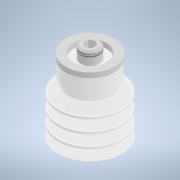
# Autodesk Inventor part: 189401 ESS-20-CS
Saved by Autodesk Inventor 2021 (Build 250183000, 183)
## iProperties
Created: 2026-04-25
Part Number: 189401 ESS-20-CS
Material: Generic
Catalog Web Link: www.3dfindit.com
Description: ESS-...-C-Suction cup complete
Vendor: FESTO
Document SubType Name: Modeling
Designer: psAdmin
Manufacturer: FESTO
Mass: 6.9 g
Surface Area: 38.5518 cm^2
Volume: 1.64725 cm^3
Density: 1 g/cm^3
Appearance: PSOLRGB-242-242-242
Category: PARTsolutions
Company: FESTO
Title: 189401 ESS-20-CS
Author: Cadenas PARTsolutions
Comments: Suction cup complete
PSOL_IDENT_0: {$CADENAS_DATA/23d-libs/festo/parts/e/ess/ess_c.prj},175 {VTYP=3D},{NB=189401 ESS-20-CS},{LINA=18940
PSOL_IDENT_1: 1 ESS-20-CS},{NN=ESS-...-C},{DATE=17.07.2025 08:23:31},{GEOMDATE=17.07.2025 08:23:17},{VERSION=},{LI
PSOL_IDENT_2: NEID=90},{WBVAR=},{WBNUMERIC=}  {NB=189401 ESS-20-CS},{LINA=189401 ESS-20-CS},{KT=2},{TNR=189401},{T
PSOL_IDENT_3: YP=ESS-20},{IDCODE=ESS-20-CS},{V=2.000},{MAT=CS},{COLOR=0.95,0.95,0.95,0.00},{MATN=15},{D1=20.000},{
PSOL_IDENT_4: D=3.000},{D2=15.000},{D3=15.500},{L1=23.000},{L2=2.400},{L3=16.400},{M=M6x1},{H=7.000},{M1=6.000},{Z
PSOL_IDENT_5: Z=0.1},{GR=4},{NENN=20},{GEO=2.000},{SDMN=20},{CNSMASSEXACT=0.00690},{GTIN=4052568042639},{REACH=Ja}
PSOL_IDENT_6: ,{REACHSVHC=Ja},{REACHHAZSUBS=7439-92-1},{REACHSCIP=a2c161a8-3d92-4cb1-8bd3-c3b2d55e9e9f},{REACHVALD
PSOL_IDENT_7: ATE=05.03.2025}
NB: 189401 ESS-20-CS
NN: ESS-...-C
NT: Suction cup complete
NBSYN: $TNR. $TYP.-$MAT.
LINA: 189401 ESS-20-CS
CATALOG: Festo
TNR: 189401
TYP: ESS-20
D1: 20
D: 3
D2: 15
D3: 15.5
L1: 23
L2: 2.4
L3: 16.4
M: M6x1
H: 7
CNSMASSEXACT: 0.0069
GTIN: 4052568042639
REACH: Yes
REACHSVHC: Yes
REACHHAZSUBS: 7439-92-1
REACHVALDATE: 05.03.2025
SUPPLIER: FESTO
ARTICLENO: 189401 ESS-20-CS
BOMINFO: 189401 ESS-20-CS
CREATOR: CADENAS GmbH
Autodesk Inventor part; units mm, degrees
sketch "Sketch_1" plane through (0, 0, 0) normal (0, 0, 1) x (1, 0, 0)
  line L0 (0, 16.0172) -> (0, 25.4)
  line L1 (0, 25.4) -> (2.3865, 25.4)
  line L2 (2.3865, 25.4) -> (3, 24.7865)
  line L3 (3, 24.7865) -> (3, 21.4)
  line L4 (3, 21.4) -> (5.25, 21.4)
  line L5 (5.25, 21.4) -> (5.25, 23)
  line L6 (5.25, 23) -> (7.75, 23)
  line L7 (7.75, 23) -> (7.75, 21.4)
  line L8 (7.75, 21.4) -> (7.25, 21.4)
  arc A0 (7.5, 21.15) -> (7.25, 21.4) centre (7.25, 21.15) ccw
  line L9 (7.5, 21.15) -> (7.5, 16.4)
  line L10 (7.5, 16.4) -> (6.75, 16.4)
  line L11 (6.75, 16.4) -> (6.75, 14.4)
  line L12 (6.75, 14.4) -> (9.5, 12.3)
  line L13 (9.5, 12.3) -> (10, 12.3)
  line L14 (10, 12.3) -> (10, 11.6333)
  line L15 (10, 11.6333) -> (9.5, 11.6333)
  line L16 (9.5, 11.6333) -> (7.2766, 10.3497)
  arc A1 (7.2766, 10.3497) -> (7.2766, 9.4837) centre (7.5266, 9.9167) ccw
  line L17 (7.2766, 9.4837) -> (9.5, 8.2)
  line L18 (9.5, 8.2) -> (10, 8.2)
  line L19 (10, 8.2) -> (10, 7.5333)
  line L20 (10, 7.5333) -> (9.5, 7.5333)
  line L21 (9.5, 7.5333) -> (7.2766, 6.2497)
  arc A2 (7.2766, 6.2497) -> (7.2766, 5.3837) centre (7.5266, 5.8167) ccw
  line L22 (7.2766, 5.3837) -> (9.5, 4.1)
  line L23 (9.5, 4.1) -> (10, 4.1)
  line L24 (10, 4.1) -> (10, 3.4333)
  line L25 (10, 3.4333) -> (9.5, 3.4333)
  line L26 (9.5, 3.4333) -> (7.4766, 2.2651)
  arc A3 (7.4766, 2.2651) -> (7.4766, 1.7455) centre (7.6266, 2.0053) ccw
  line L27 (7.4766, 1.7455) -> (10.1439, 0.2056)
  line L28 (10.1439, 0.2056) -> (10, 0)
  line L29 (10, 0) -> (6.5766, 1.9765)
  line L30 (6.5766, 1.9765) -> (9.6774, 3.7667)
  line L31 (9.6774, 3.7667) -> (6.1266, 5.8167)
  line L32 (6.1266, 5.8167) -> (9.6774, 7.8667)
  line L33 (9.6774, 7.8667) -> (6.1266, 9.9167)
  line L34 (6.1266, 9.9167) -> (9.6373, 11.9435)
  line L35 (9.6373, 11.9435) -> (6.6286, 14.241)
  line L36 (6.6286, 14.241) -> (0, 16.0172)
  line L37 (0, 16.0172) -> (0, 25.4)
  constraints: 76 end point, 8 point on circle, 4 centre point
revolve "Revolution1" add sketch "Sketch_1" angle 360 about axis through (0, 16.0172, 0) along (0, 1, 0)
thread "Thread1" size "M6x1" class "6g" standard "ISO Metric profile" length 1.0365
sketch "Sketch_2" plane through (0, 25.4, 0) normal (0, 1, 0) x (1, 0, 0)
  line L0 (-1.5, -0.866) -> (0, -1.7321)
  line L1 (0, -1.7321) -> (1.5, -0.866)
  line L2 (1.5, -0.866) -> (1.5, 0.866)
  line L3 (1.5, 0.866) -> (0, 1.7321)
  line L4 (0, 1.7321) -> (-1.5, 0.866)
  line L5 (-1.5, 0.866) -> (-1.5, -0.866)
  constraints: 12 end point
extrude "Extrusion1" cut sketch "Sketch_2" against normal blind 23
ref_plane "Halter_XY" through (0, 21.4, 0) normal (0, 1, 0) x (1, 0, 0)
ref_plane "Halter_YZ" through (0, 21.4, 0) normal (1, 0, 0) x (0, 0, -1)
ref_plane "Halter_ZX" through (0, 21.4, 0) normal (0, 0, -1) x (0, 1, 0)
ref_plane "Halter1_XY" through (0, 23, 0) normal (0, 1, 0) x (1, 0, 0)
ref_plane "Halter1_YZ" through (0, 23, 0) normal (1, 0, 0) x (0, 0, -1)
ref_plane "Halter1_ZX" through (0, 23, 0) normal (0, 0, -1) x (0, 1, 0)
ref_plane "START_XY" through (0, 0, 0) normal (0, 1, 0) x (1, 0, 0)
ref_plane "START_YZ" through (0, 0, 0) normal (1, 0, 0) x (0, 0, -1)
ref_plane "START_ZX" through (0, 0, 0) normal (0, 0, -1) x (0, 1, 0)
body "Solid1"
